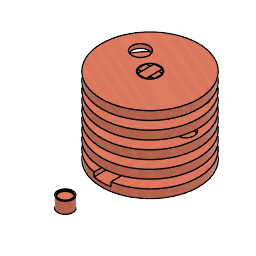
NestorBrinquedo_TorreLabirinto_MariaCarrilho (Autodesk Fusion 360 design; units mm, degrees)
Autodesk Fusion 360 part; units mm, degrees
note: some values were not read from the file. Set by a fixed rule: which sketch regions a step uses; which face or edge a step refers to.
sketch "Esboço1" plane through (0, 0, 0) normal (0, 1, 0) x (1, 0, 0) in component "Camada_2"
  circle A0 centre (0, 0) radius 11.3803
  line L0 (10, 5) -> (-10, 5)
  line L1 (-10, 5) -> (-10, -5)
  line L2 (-10, -5) -> (10, -5)
  line L3 (10, -5) -> (10, 5)
  line L4 (10, 5) -> (-10, -5) construction
  line L5 (-10, 5) -> (10, -5) construction
  line L6 (5, 10) -> (-5, 10)
  line L7 (-5, 10) -> (-5, -10)
  line L8 (-5, -10) -> (5, -10)
  line L9 (5, -10) -> (5, 10)
  line L10 (5, 10) -> (-5, -10) construction
  line L11 (-5, 10) -> (5, -10) construction
  spline S0 degree 3 poles (41.2019, -26.9625) (41.0951, -21.5825) (35.0181, -15.8495) (34.4042, -15.28) knots 0 0 0 0 1 1 1 1
  spline S1 degree 2 poles (34.4042, -15.28) (29.2732, -10.5317) (18.8986, -4.6652) knots 0 0 0 1 1 1
  spline S2 degree 3 poles (18.8986, -4.6652) (18.4699, -4.2135) (17.9685, -3.7052) (17.3893, -2.8657) knots 0 0 0 0 1 1 1 1
  spline S3 degree 3 poles (2.7382, 14.1172) (2.5277, 14.3871) (2.2815, 14.7312) (2.0205, 15.1909) knots 0 0 0 0 1 1 1 1
  spline S4 degree 2 poles (2.0205, 15.1909) (0.8016, 17.3352) (0.4873, 20.138) knots 0 0 0 1 1 1
  spline S5 degree 3 poles (0.4873, 20.138) (0.4873, 20.1409) (0.4873, 20.2892) (0.2856, 21.4578) knots 0 0 0 0 1 1 1 1
  spline S6 degree 3 poles (0.2856, 21.4578) (-0.9393, 28.5165) (0.2885, 39.1461) (4.4259, 42.7141) knots 0 0 0 0 1 1 1 1
  spline S7 degree 3 poles (4.4259, 42.7141) (4.7877, 43.0255) (5.805, 43.8293) (6.2617, 45.2291) knots 0 0 0 0 1 1 1 1
  spline S8 degree 3 poles (6.2617, 45.2291) (6.8045, 46.8841) (6.499, 49.153) (5.2978, 49.7135) knots 0 0 0 0 1 1 1 1
  spline S9 degree 3 poles (5.2978, 49.7135) (4.3962, 50.1347) (3.2603, 49.4674) (2.7502, 49.1619) knots 0 0 0 0 1 1 1 1
  spline S10 degree 3 poles (2.7502, 49.1619) (-1.8558, 46.3799) (-3.7807, 38.2505) (-3.9675, 37.4319) knots 0 0 0 0 1 1 1 1
  spline S11 degree 2 poles (-3.9675, 37.4319) (-5.5157, 30.6164) (-5.4059, 18.6966) knots 0 0 0 1 1 1
  spline S12 degree 3 poles (-5.4059, 18.6966) (-5.4952, 18.0832) (-5.5848, 17.3707) (-5.8856, 16.4) knots 0 0 0 0 1 1 1 1
  spline S13 degree 3 poles (-13.5935, -4.6916) (-13.724, -5.006) (-13.9019, -5.3916) (-14.1689, -5.8454) knots 0 0 0 0 1 1 1 1
  spline S14 degree 2 poles (-14.1689, -5.8454) (-15.4145, -7.9689) (-17.6834, -9.6476) knots 0 0 0 1 1 1
  line L12 (-17.6834, -9.6476) -> (-17.6861, -9.6476)
  spline S15 degree 2 poles (-17.6861, -9.6476) (-17.8166, -9.7217) (-18.7241, -10.481) knots 0 0 0 1 1 1
  spline S16 degree 3 poles (-18.7241, -10.481) (-24.2258, -15.0721) (-34.0457, -19.3222) (-39.2034, -17.5249) knots 0 0 0 0 1 1 1 1
  spline S17 degree 3 poles (-39.2034, -17.5249) (-39.6571, -17.3677) (-40.8583, -16.8872) (-42.3027, -17.1927) knots 0 0 0 0 1 1 1 1
  spline S18 degree 3 poles (-42.3027, -17.1927) (-44.0081, -17.5486) (-45.8172, -18.9485) (-45.7016, -20.2683) knots 0 0 0 0 1 1 1 1
  spline S19 degree 3 poles (-45.7016, -20.2683) (-45.6156, -21.2619) (-44.4707, -21.9114) (-43.9487, -22.1991) knots 0 0 0 0 1 1 1 1
  spline S20 degree 3 poles (-43.9487, -22.1991) (-39.239, -24.7972) (-31.2341, -22.4007) (-30.4333, -22.1516) knots 0 0 0 0 1 1 1 1
  spline S21 degree 2 poles (-30.4333, -22.1516) (-23.7572, -20.0844) (-13.4894, -14.0311) knots 0 0 0 1 1 1
  spline S22 degree 3 poles (-13.4894, -14.0311) (-12.9117, -13.8003) (-12.2543, -13.5185) (-11.2626, -13.2872) knots 0 0 0 0 1 1 1 1
  spline S23 degree 3 poles (10.8582, -9.4283) (11.1963, -9.3809) (11.6175, -9.3423) (12.1484, -9.3453) knots 0 0 0 0 1 1 1 1
  spline S24 degree 2 poles (12.1484, -9.3453) (14.61, -9.3631) (17.1962, -10.4931) knots 0 0 0 1 1 1
  line L13 (17.1962, -10.4931) -> (17.1992, -10.4931)
  spline S25 degree 2 poles (17.1992, -10.4931) (17.3297, -10.5673) (18.4419, -10.9765) knots 0 0 0 1 1 1
  spline S26 degree 3 poles (18.4419, -10.9765) (25.1685, -13.4441) (33.7576, -19.8237) (34.7808, -25.1889) knots 0 0 0 0 1 1 1 1
  spline S27 degree 3 poles (34.7808, -25.1889) (34.8698, -25.6605) (35.0566, -26.9418) (36.0413, -28.0391) knots 0 0 0 0 1 1 1 1
  spline S28 degree 3 poles (36.0413, -28.0391) (37.2039, -29.3352) (39.3216, -30.2042) (40.4071, -29.4449) knots 0 0 0 0 1 1 1 1
  spline S29 degree 3 poles (40.4071, -29.4449) (41.2227, -28.8755) (41.2138, -27.5587) (41.2019, -26.9625) knots 0 0 0 0 1 1 1 1
  circle A1 centre (0, 0) radius 57
  circle A2 centre (0, 0) radius 52
  line L14 (0, 57) -> (0, -57) construction
  circle A3 centre (0, 0) radius 11.1803 construction
  circle A4 centre (0, 0) radius 14.3803
  line L15 (-11.2626, -13.2872) -> (-7.3325, -12.3705)
  line L16 (17.3893, -2.8657) -> (14.2878, 1.6289)
  line L17 (-5.8856, 16.4) -> (-7.0909, 12.5106)
  line L18 (0, -52) -> (45.0333, 26) construction
  line L19 (45.0333, 26) -> (-45.0333, 26) construction
  line L20 (-45.0333, 26) -> (0, -52) construction
  line L21 (0, 0) -> (-45.0333, 26) construction
  line L22 (0, 0) -> (45.0333, 26) construction
  circle A5 centre (0, -31) radius 10
  circle A6 centre (-21.114, 12.1902) radius 10
  circle A7 centre (36.3731, 21) radius 10
  line L23 (0, -14.3803) -> (0, -52) construction
  point P0 (-0.2433, -0.1238)
  dimension "d39" = 10
  dimension "d40" = 10
  dimension "d41" = 20
  dimension "d42" = 20
  dimension "d43" = 0.2
  dimension "d45" = 114
  dimension "d46" = 5
  dimension "d47" = 3
  dimension "d48" = 20
  dimension "d49" = 20
  dimension "d50" = 20
  dimension "d51" = 31
  constraint coincident A0.centre A1.centre
  constraint horizontal L0
  constraint perpendicular L0 L1
  constraint parallel L0 L2
  constraint parallel L1 L3
  constraint coincident L4 A0.centre
  constraint coincident L5 A0.centre
  constraint horizontal L6
  constraint perpendicular L6 L7
  constraint parallel L6 L8
  constraint parallel L7 L9
  constraint coincident L10 A0.centre
  constraint coincident L11 A0.centre
  constraint concentric A0 A1
  constraint concentric A0 A2
  constraint coincident A1 L14.start
  constraint coincident A1 L14.end
  constraint vertical L14
  constraint coincident A0.centre L14
  constraint concentric A1 A3
  constraint coincident L6.start A3
  constraint concentric A0 A4
  constraint coincident S13.start A4
  constraint coincident S3.start A4
  constraint coincident S23.start A4
  constraint coincident A4 L15.end
  constraint coincident A4 L16.end
  constraint coincident A4 L17.end
  constraint coincident L14 L18.start
  constraint coincident A2 L18.start
  constraint coincident L21 A6.centre
  constraint coincident L22 A7.centre
  constraint tangent A2 A7
  constraint tangent A4 A6
  constraint coincident L14 L23.start
  constraint coincident A4 L23.start
  constraint coincident A5.centre L23
  measures "d39" distance of L0 L2
  measures "d40" distance of L7 L9
  measures "d41" distance of L1 L3
  measures "d42" distance of L6 L8
  measures "d43" distance of A0 A3
  measures "d45" diameter of A1
  measures "d46" distance of A1 A2
  measures "d47" distance of A0 A4
  measures "d48" diameter of A6
  measures "d49" diameter of A7
  measures "d50" diameter of A5
  measures "d51" distance of A0.centre A5.centre
sketch "Esboço1 (2)" plane through (0, 0, 0) normal (0, 1, 0) x (1, 0, 0) in component "Camada_3"
  line L0 (-5, 10) -> (-5, -10)
  line L1 (5, 10) -> (-5, 10)
  line L2 (-5, 10) -> (5, -10) construction
  line L3 (5, 10) -> (-5, -10) construction
  line L4 (5, -10) -> (5, 10)
  line L5 (-5, -10) -> (5, -10)
  line L6 (-10, -5) -> (10, -5)
  line L7 (-10, 5) -> (10, -5) construction
  line L8 (10, -5) -> (10, 5)
  line L9 (10, 5) -> (-10, -5) construction
  line L10 (10, 5) -> (-10, 5)
  line L11 (-10, 5) -> (-10, -5)
  circle A0 centre (0, 0) radius 11.1803 construction
  circle A1 centre (0, 0) radius 11.3803
  circle A2 centre (0, 0) radius 14.3803
  circle A3 centre (0, 0) radius 57
  circle A4 centre (0, 0) radius 52
  line L12 (-5.8856, 16.4) -> (-7.0909, 12.5106)
  spline S0 degree 3 poles (-5.4059, 18.6966) (-5.4952, 18.0832) (-5.5848, 17.3707) (-5.8856, 16.4) knots 0 0 0 0 1 1 1 1
  spline S1 degree 2 poles (-3.9675, 37.4319) (-5.5157, 30.6164) (-5.4059, 18.6966) knots 0 0 0 1 1 1
  spline S2 degree 3 poles (0.4873, 20.138) (0.4873, 20.1409) (0.4873, 20.2892) (0.2856, 21.4578) knots 0 0 0 0 1 1 1 1
  spline S3 degree 2 poles (2.0205, 15.1909) (0.8016, 17.3352) (0.4873, 20.138) knots 0 0 0 1 1 1
  spline S4 degree 3 poles (2.7382, 14.1172) (2.5277, 14.3871) (2.2815, 14.7312) (2.0205, 15.1909) knots 0 0 0 0 1 1 1 1
  spline S5 degree 3 poles (0.2856, 21.4578) (-0.9393, 28.5165) (0.2885, 39.1461) (4.4259, 42.7141) knots 0 0 0 0 1 1 1 1
  spline S6 degree 3 poles (2.7502, 49.1619) (-1.8558, 46.3799) (-3.7807, 38.2505) (-3.9675, 37.4319) knots 0 0 0 0 1 1 1 1
  spline S7 degree 3 poles (5.2978, 49.7135) (4.3962, 50.1347) (3.2603, 49.4674) (2.7502, 49.1619) knots 0 0 0 0 1 1 1 1
  spline S8 degree 3 poles (6.2617, 45.2291) (6.8045, 46.8841) (6.499, 49.153) (5.2978, 49.7135) knots 0 0 0 0 1 1 1 1
  spline S9 degree 3 poles (4.4259, 42.7141) (4.7877, 43.0255) (5.805, 43.8293) (6.2617, 45.2291) knots 0 0 0 0 1 1 1 1
  line L13 (0, -14.3803) -> (0, -52) construction
  line L14 (0, 57) -> (0, -57) construction
  spline S10 degree 3 poles (-6.262, -45.2316) (-6.8065, -46.8864) (-6.4987, -49.1531) (-5.2979, -49.7129) knots 0 0 0 0 1 1 1 1
  line L15 (-6.262, -45.2316) -> (-6.8065, -46.8864) construction
  line L16 (-6.8065, -46.8864) -> (-6.4987, -49.1531) construction
  line L17 (-6.4987, -49.1531) -> (-5.2979, -49.7129) construction
  spline S11 degree 3 poles (-5.2979, -49.7129) (-4.3945, -50.1352) (-3.2596, -49.4685) (-2.7494, -49.1603) knots 0 0 0 0 1 1 1 1
  line L18 (-5.2979, -49.7129) -> (-4.3945, -50.1352) construction
  line L19 (-4.3945, -50.1352) -> (-3.2596, -49.4685) construction
  line L20 (-3.2596, -49.4685) -> (-2.7494, -49.1603) construction
  spline S12 degree 3 poles (-2.7494, -49.1603) (1.8555, -46.3805) (3.7826, -38.2499) (3.9672, -37.4318) knots 0 0 0 0 1 1 1 1
  line L21 (-2.7494, -49.1603) -> (1.8555, -46.3805) construction
  line L22 (1.8555, -46.3805) -> (3.7826, -38.2499) construction
  line L23 (3.7826, -38.2499) -> (3.9672, -37.4318) construction
  spline S13 degree 3 poles (-4.4247, -42.7135) (-4.7877, -43.0279) (-5.8044, -43.8279) (-6.262, -45.2316) knots 0 0 0 0 1 1 1 1
  line L24 (-4.4247, -42.7135) -> (-4.7877, -43.0279) construction
  line L25 (-4.7877, -43.0279) -> (-5.8044, -43.8279) construction
  line L26 (-5.8044, -43.8279) -> (-6.262, -45.2316) construction
  spline S14 degree 3 poles (-0.2852, -21.456) (0.94, -28.5162) (-0.2894, -39.1456) (-4.4247, -42.7135) knots 0 0 0 0 1 1 1 1
  line L27 (-0.2852, -21.456) -> (0.94, -28.5162) construction
  line L28 (0.94, -28.5162) -> (-0.2894, -39.1456) construction
  line L29 (-0.2894, -39.1456) -> (-4.4247, -42.7135) construction
  spline S15 degree 2 poles (3.9672, -37.4318) (5.515, -30.6165) (5.4066, -18.6977) knots 0 0 0 1 1 1
  line L30 (3.9672, -37.4318) -> (5.515, -30.6165) construction
  line L31 (5.515, -30.6165) -> (5.4066, -18.6977) construction
  spline S16 degree 2 poles (-2.0222, -15.1933) (-0.806, -17.3338) (-0.4867, -20.1381) knots 0 0 0 1 1 1
  line L32 (-2.0222, -15.1933) -> (-0.806, -17.3338) construction
  line L33 (-0.806, -17.3338) -> (-0.4867, -20.1381) construction
  spline S17 degree 2 poles (-0.4867, -20.1381) (-0.4878, -20.2976) (-0.2852, -21.456) knots 0 0 0 1 1 1
  line L34 (-0.4867, -20.1381) -> (-0.4878, -20.2976) construction
  line L35 (-0.4878, -20.2976) -> (-0.2852, -21.456) construction
  spline S18 degree 3 poles (5.4066, -18.6977) (5.4956, -18.082) (5.5803, -17.3718) (5.8758, -16.3973) knots 0 0 0 0 1 1 1 1
  line L36 (5.4066, -18.6977) -> (5.4956, -18.082) construction
  line L37 (5.4956, -18.082) -> (5.5803, -17.3718) construction
  line L38 (5.5803, -17.3718) -> (5.8758, -16.3973) construction
  line L39 (5.8758, -16.3973) -> (7.0469, -12.5353)
  spline S19 degree 3 poles (-2.7337, -14.1181) (-2.5266, -14.3883) (-2.2817, -14.7352) (-2.0222, -15.1933) knots 0 0 0 0 1 1 1 1
  line L40 (-2.7337, -14.1181) -> (-2.5266, -14.3883) construction
  line L41 (-2.5266, -14.3883) -> (-2.2817, -14.7352) construction
  line L42 (-2.2817, -14.7352) -> (-2.0222, -15.1933) construction
  line L43 (-57, 0) -> (57, 0) construction
  circle A5 centre (-24.3803, 0) radius 10
  circle A6 centre (42, 0) radius 10
  dimension "d52" = 20
  dimension "d53" = 20
  constraint coincident A3 L43.start
  constraint coincident A3 L43.end
  constraint perpendicular L8 L43
  constraint coincident L43 A0.centre
  constraint coincident L43 A5.centre
  constraint coincident L43 A6.centre
  constraint tangent A2 A5
  constraint tangent A4 A6
  constraint coincident A2 S19.start
  constraint coincident A2 L39.end
  constraint coincident S16.end L33.end
  measures "d52" diameter of A5
  measures "d53" diameter of A6
sketch "Esboço1 (3)" plane through (0, 0, 0) normal (0, 1, 0) x (1, 0, 0) in component "Camada_4"
  circle A0 centre (0, 0) radius 57
  circle A1 centre (0, 0) radius 52
  line L0 (-5.8856, 16.4) -> (-7.0909, 12.5106)
  spline S0 degree 3 poles (-5.4059, 18.6966) (-5.4952, 18.0832) (-5.5848, 17.3707) (-5.8856, 16.4) knots 0 0 0 0 1 1 1 1
  spline S1 degree 2 poles (-3.9675, 37.4319) (-5.5157, 30.6164) (-5.4059, 18.6966) knots 0 0 0 1 1 1
  spline S2 degree 3 poles (2.7502, 49.1619) (-1.8558, 46.3799) (-3.7807, 38.2505) (-3.9675, 37.4319) knots 0 0 0 0 1 1 1 1
  spline S3 degree 3 poles (5.2978, 49.7135) (4.3962, 50.1347) (3.2603, 49.4674) (2.7502, 49.1619) knots 0 0 0 0 1 1 1 1
  spline S4 degree 3 poles (6.2617, 45.2291) (6.8045, 46.8841) (6.499, 49.153) (5.2978, 49.7135) knots 0 0 0 0 1 1 1 1
  spline S5 degree 3 poles (4.4259, 42.7141) (4.7877, 43.0255) (5.805, 43.8293) (6.2617, 45.2291) knots 0 0 0 0 1 1 1 1
  spline S6 degree 3 poles (0.2856, 21.4578) (-0.9393, 28.5165) (0.2885, 39.1461) (4.4259, 42.7141) knots 0 0 0 0 1 1 1 1
  spline S7 degree 2 poles (2.0205, 15.1909) (0.8016, 17.3352) (0.4873, 20.138) knots 0 0 0 1 1 1
  spline S8 degree 3 poles (0.4873, 20.138) (0.4873, 20.1409) (0.4873, 20.2892) (0.2856, 21.4578) knots 0 0 0 0 1 1 1 1
  spline S9 degree 3 poles (2.7382, 14.1172) (2.5277, 14.3871) (2.2815, 14.7312) (2.0205, 15.1909) knots 0 0 0 0 1 1 1 1
  circle A2 centre (0, 0) radius 14.3803
  circle A3 centre (0, 0) radius 11.3803
  circle A4 centre (0, 0) radius 11.1803 construction
  line L1 (10, 5) -> (-10, -5) construction
  line L2 (-10, 5) -> (-10, -5)
  line L3 (-10, 5) -> (10, -5) construction
  line L4 (10, 5) -> (-10, 5)
  line L5 (-5, 10) -> (-5, -10)
  line L6 (5, 10) -> (-5, 10)
  line L7 (-5, 10) -> (5, -10) construction
  line L8 (5, 10) -> (-5, -10) construction
  line L9 (5, -10) -> (5, 10)
  line L10 (-10, -5) -> (10, -5)
  line L11 (-5, -10) -> (5, -10)
  line L12 (10, -5) -> (10, 5)
  line L13 (0, 57) -> (0, -57) construction
  circle A5 centre (0, -31) radius 10
sketch "Esboço1 (4)" plane through (0, 0, 0) normal (0, 1, 0) x (1, 0, 0) in component "Base"
  circle A0 centre (0, 0) radius 57
  circle A1 centre (0, 0) radius 52
  circle A2 centre (0, 0) radius 14.3803
  circle A3 centre (0, 0) radius 11.3803
  circle A4 centre (0, 0) radius 11.1803 construction
  line L0 (-10, -5) -> (10, -5)
  line L1 (-10, 5) -> (-10, -5)
  line L2 (10, 5) -> (-10, -5) construction
  line L3 (-10, 5) -> (10, -5) construction
  line L4 (10, 5) -> (-10, 5)
  line L5 (-5, 10) -> (-5, -10)
  line L6 (5, 10) -> (-5, 10)
  line L7 (5, -10) -> (5, 10)
  line L8 (5, 10) -> (-5, -10) construction
  line L9 (-5, 10) -> (5, -10) construction
  line L10 (10, -5) -> (10, 5)
  line L11 (-5, -10) -> (5, -10)
  circle A5 centre (0, -31) radius 10
  line L12 (0, 57) -> (0, -57) construction
  line L13 (-10, -31) -> (10, -31) construction
  line L14 (-10, -31) -> (10, -31) construction
  line L15 (10, -31) -> (10, -57)
  line L16 (10, -57) -> (-10, -57)
  line L17 (-10, -57) -> (-10, -31)
  constraint coincident A5 L13.start
  constraint coincident A5 L13.end
  constraint perpendicular L12 L13
  constraint perpendicular L14 L15
  constraint parallel L14 L16
  constraint parallel L15 L17
  constraint coincident L12.end L16
  constraint tangent A5 L17
sketch "Esboço1 (5)" plane through (0, 0, 0) normal (0, 1, 0) x (1, 0, 0) in component "Tampa_cam1"
  circle A0 centre (0, 0) radius 57
  circle A1 centre (0, 0) radius 52
  spline S0 degree 3 poles (5.2978, 49.7135) (4.3962, 50.1347) (3.2603, 49.4674) (2.7502, 49.1619) knots 0 0 0 0 1 1 1 1
  spline S1 degree 3 poles (6.2617, 45.2291) (6.8045, 46.8841) (6.499, 49.153) (5.2978, 49.7135) knots 0 0 0 0 1 1 1 1
  spline S2 degree 3 poles (4.4259, 42.7141) (4.7877, 43.0255) (5.805, 43.8293) (6.2617, 45.2291) knots 0 0 0 0 1 1 1 1
  spline S3 degree 3 poles (0.2856, 21.4578) (-0.9393, 28.5165) (0.2885, 39.1461) (4.4259, 42.7141) knots 0 0 0 0 1 1 1 1
  spline S4 degree 3 poles (2.7502, 49.1619) (-1.8558, 46.3799) (-3.7807, 38.2505) (-3.9675, 37.4319) knots 0 0 0 0 1 1 1 1
  spline S5 degree 2 poles (-3.9675, 37.4319) (-5.5157, 30.6164) (-5.4059, 18.6966) knots 0 0 0 1 1 1
  spline S6 degree 3 poles (-5.4059, 18.6966) (-5.4952, 18.0832) (-5.5848, 17.3707) (-5.8856, 16.4) knots 0 0 0 0 1 1 1 1
  line L0 (-5.8856, 16.4) -> (-7.0909, 12.5106)
  spline S7 degree 2 poles (2.0205, 15.1909) (0.8016, 17.3352) (0.4873, 20.138) knots 0 0 0 1 1 1
  spline S8 degree 3 poles (0.4873, 20.138) (0.4873, 20.1409) (0.4873, 20.2892) (0.2856, 21.4578) knots 0 0 0 0 1 1 1 1
  spline S9 degree 3 poles (2.7382, 14.1172) (2.5277, 14.3871) (2.2815, 14.7312) (2.0205, 15.1909) knots 0 0 0 0 1 1 1 1
  circle A2 centre (0, 0) radius 14.3803
  circle A3 centre (0, 0) radius 11.3803
  circle A4 centre (0, 0) radius 11.1803 construction
  line L1 (5, 10) -> (-5, 10)
  line L2 (-5, 10) -> (-5, -10)
  line L3 (-5, -10) -> (5, -10)
  line L4 (5, -10) -> (5, 10)
  line L5 (10, 5) -> (-10, 5)
  line L6 (-10, 5) -> (-10, -5)
  line L7 (-10, -5) -> (10, -5)
  line L8 (10, -5) -> (10, 5)
  line L9 (-10, 5) -> (10, -5) construction
  line L10 (10, 5) -> (-10, -5) construction
  line L11 (5, 10) -> (-5, -10) construction
  line L12 (-5, 10) -> (5, -10) construction
  line L13 (0, 57) -> (0, -57) construction
  line L14 (-57, 0) -> (57, 0) construction
  spline S10 degree 3 poles (-5.2979, -49.7129) (-4.3945, -50.1352) (-3.2596, -49.4685) (-2.7494, -49.1603) knots 0 0 0 0 1 1 1 1
  spline S11 degree 3 poles (-6.262, -45.2316) (-6.8065, -46.8864) (-6.4987, -49.1531) (-5.2979, -49.7129) knots 0 0 0 0 1 1 1 1
  spline S12 degree 3 poles (-4.4247, -42.7135) (-4.7877, -43.0279) (-5.8044, -43.8279) (-6.262, -45.2316) knots 0 0 0 0 1 1 1 1
  spline S13 degree 3 poles (-0.2852, -21.456) (0.94, -28.5162) (-0.2894, -39.1456) (-4.4247, -42.7135) knots 0 0 0 0 1 1 1 1
  spline S14 degree 3 poles (-2.7494, -49.1603) (1.8555, -46.3805) (3.7826, -38.2499) (3.9672, -37.4318) knots 0 0 0 0 1 1 1 1
  spline S15 degree 2 poles (3.9672, -37.4318) (5.515, -30.6165) (5.4066, -18.6977) knots 0 0 0 1 1 1
  spline S16 degree 2 poles (-0.4867, -20.1381) (-0.4878, -20.2976) (-0.2852, -21.456) knots 0 0 0 1 1 1
  spline S17 degree 2 poles (-2.0222, -15.1933) (-0.806, -17.3338) (-0.4867, -20.1381) knots 0 0 0 1 1 1
  spline S18 degree 3 poles (5.4066, -18.6977) (5.4956, -18.082) (5.5803, -17.3718) (5.8758, -16.3973) knots 0 0 0 0 1 1 1 1
  line L15 (5.8758, -16.3973) -> (7.0469, -12.5353)
  spline S19 degree 3 poles (-2.7337, -14.1181) (-2.5266, -14.3883) (-2.2817, -14.7352) (-2.0222, -15.1933) knots 0 0 0 0 1 1 1 1
  spline S20 degree 2 poles (-37.4319, -3.9675) (-30.6164, -5.5157) (-18.6966, -5.4059) knots 0 0 0 1 1 1
  line L16 (-37.4319, -3.9675) -> (-30.6164, -5.5157) construction
  line L17 (-30.6164, -5.5157) -> (-18.6966, -5.4059) construction
  spline S21 degree 3 poles (-18.6966, -5.4059) (-18.0832, -5.4952) (-17.3707, -5.5848) (-16.4, -5.8856) knots 0 0 0 0 1 1 1 1
  line L18 (-18.6966, -5.4059) -> (-18.0832, -5.4952) construction
  line L19 (-18.0832, -5.4952) -> (-17.3707, -5.5848) construction
  line L20 (-17.3707, -5.5848) -> (-16.4, -5.8856) construction
  line L21 (-16.4, -5.8856) -> (-12.5106, -7.0909)
  spline S22 degree 2 poles (-15.1909, 2.0205) (-17.3352, 0.8016) (-20.138, 0.4873) knots 0 0 0 1 1 1
  line L22 (-15.1909, 2.0205) -> (-17.3352, 0.8016) construction
  line L23 (-17.3352, 0.8016) -> (-20.138, 0.4873) construction
  spline S23 degree 3 poles (-14.1172, 2.7382) (-14.3871, 2.5277) (-14.7312, 2.2815) (-15.1909, 2.0205) knots 0 0 0 0 1 1 1 1
  line L24 (-14.1172, 2.7382) -> (-14.3871, 2.5277) construction
  line L25 (-14.3871, 2.5277) -> (-14.7312, 2.2815) construction
  line L26 (-14.7312, 2.2815) -> (-15.1909, 2.0205) construction
  spline S24 degree 3 poles (-21.4578, 0.2856) (-28.5165, -0.9393) (-39.1461, 0.2885) (-42.7141, 4.4259) knots 0 0 0 0 1 1 1 1
  line L27 (-21.4578, 0.2856) -> (-28.5165, -0.9393) construction
  line L28 (-28.5165, -0.9393) -> (-39.1461, 0.2885) construction
  line L29 (-39.1461, 0.2885) -> (-42.7141, 4.4259) construction
  spline S25 degree 3 poles (-20.138, 0.4873) (-20.1409, 0.4873) (-20.2892, 0.4873) (-21.4578, 0.2856) knots 0 0 0 0 1 1 1 1
  line L30 (-20.138, 0.4873) -> (-20.1409, 0.4873) construction
  line L31 (-20.1409, 0.4873) -> (-20.2892, 0.4873) construction
  line L32 (-20.2892, 0.4873) -> (-21.4578, 0.2856) construction
  spline S26 degree 3 poles (-49.1619, 2.7502) (-46.3799, -1.8558) (-38.2505, -3.7807) (-37.4319, -3.9675) knots 0 0 0 0 1 1 1 1
  line L33 (-49.1619, 2.7502) -> (-46.3799, -1.8558) construction
  line L34 (-46.3799, -1.8558) -> (-38.2505, -3.7807) construction
  line L35 (-38.2505, -3.7807) -> (-37.4319, -3.9675) construction
  spline S27 degree 3 poles (-49.7135, 5.2978) (-50.1347, 4.3962) (-49.4674, 3.2603) (-49.1619, 2.7502) knots 0 0 0 0 1 1 1 1
  line L36 (-49.7135, 5.2978) -> (-50.1347, 4.3962) construction
  line L37 (-50.1347, 4.3962) -> (-49.4674, 3.2603) construction
  line L38 (-49.4674, 3.2603) -> (-49.1619, 2.7502) construction
  spline S28 degree 3 poles (-45.2291, 6.2617) (-46.8841, 6.8045) (-49.153, 6.499) (-49.7135, 5.2978) knots 0 0 0 0 1 1 1 1
  line L39 (-45.2291, 6.2617) -> (-46.8841, 6.8045) construction
  line L40 (-46.8841, 6.8045) -> (-49.153, 6.499) construction
  line L41 (-49.153, 6.499) -> (-49.7135, 5.2978) construction
  spline S29 degree 3 poles (-42.7141, 4.4259) (-43.0255, 4.7877) (-43.8293, 5.805) (-45.2291, 6.2617) knots 0 0 0 0 1 1 1 1
  line L42 (-42.7141, 4.4259) -> (-43.0255, 4.7877) construction
  line L43 (-43.0255, 4.7877) -> (-43.8293, 5.805) construction
  line L44 (-43.8293, 5.805) -> (-45.2291, 6.2617) construction
  spline S30 degree 3 poles (20.138, -0.4873) (20.1409, -0.4873) (20.2892, -0.4873) (21.4578, -0.2856) knots 0 0 0 0 1 1 1 1
  line L45 (20.138, -0.4873) -> (20.1409, -0.4873) construction
  line L46 (20.1409, -0.4873) -> (20.2892, -0.4873) construction
  line L47 (20.2892, -0.4873) -> (21.4578, -0.2856) construction
  spline S31 degree 2 poles (15.1909, -2.0205) (17.3352, -0.8016) (20.138, -0.4873) knots 0 0 0 1 1 1
  line L48 (15.1909, -2.0205) -> (17.3352, -0.8016) construction
  line L49 (17.3352, -0.8016) -> (20.138, -0.4873) construction
  spline S32 degree 3 poles (45.2291, -6.2617) (46.8841, -6.8045) (49.153, -6.499) (49.7135, -5.2978) knots 0 0 0 0 1 1 1 1
  line L50 (45.2291, -6.2617) -> (46.8841, -6.8045) construction
  line L51 (46.8841, -6.8045) -> (49.153, -6.499) construction
  line L52 (49.153, -6.499) -> (49.7135, -5.2978) construction
  spline S33 degree 3 poles (49.7135, -5.2978) (50.1347, -4.3962) (49.4674, -3.2603) (49.1619, -2.7502) knots 0 0 0 0 1 1 1 1
  line L53 (49.7135, -5.2978) -> (50.1347, -4.3962) construction
  line L54 (50.1347, -4.3962) -> (49.4674, -3.2603) construction
  line L55 (49.4674, -3.2603) -> (49.1619, -2.7502) construction
  spline S34 degree 3 poles (42.7141, -4.4259) (43.0255, -4.7877) (43.8293, -5.805) (45.2291, -6.2617) knots 0 0 0 0 1 1 1 1
  line L56 (42.7141, -4.4259) -> (43.0255, -4.7877) construction
  line L57 (43.0255, -4.7877) -> (43.8293, -5.805) construction
  line L58 (43.8293, -5.805) -> (45.2291, -6.2617) construction
  line L59 (16.4, 5.8856) -> (12.5106, 7.0909)
  spline S35 degree 2 poles (37.4319, 3.9675) (30.6164, 5.5157) (18.6966, 5.4059) knots 0 0 0 1 1 1
  line L60 (37.4319, 3.9675) -> (30.6164, 5.5157) construction
  line L61 (30.6164, 5.5157) -> (18.6966, 5.4059) construction
  spline S36 degree 3 poles (49.1619, -2.7502) (46.3799, 1.8558) (38.2505, 3.7807) (37.4319, 3.9675) knots 0 0 0 0 1 1 1 1
  line L62 (49.1619, -2.7502) -> (46.3799, 1.8558) construction
  line L63 (46.3799, 1.8558) -> (38.2505, 3.7807) construction
  line L64 (38.2505, 3.7807) -> (37.4319, 3.9675) construction
  spline S37 degree 3 poles (14.1172, -2.7382) (14.3871, -2.5277) (14.7312, -2.2815) (15.1909, -2.0205) knots 0 0 0 0 1 1 1 1
  line L65 (14.1172, -2.7382) -> (14.3871, -2.5277) construction
  line L66 (14.3871, -2.5277) -> (14.7312, -2.2815) construction
  line L67 (14.7312, -2.2815) -> (15.1909, -2.0205) construction
  spline S38 degree 3 poles (18.6966, 5.4059) (18.0832, 5.4952) (17.3707, 5.5848) (16.4, 5.8856) knots 0 0 0 0 1 1 1 1
  line L68 (18.6966, 5.4059) -> (18.0832, 5.4952) construction
  line L69 (18.0832, 5.4952) -> (17.3707, 5.5848) construction
  line L70 (17.3707, 5.5848) -> (16.4, 5.8856) construction
  spline S39 degree 3 poles (21.4578, -0.2856) (28.5165, 0.9393) (39.1461, -0.2885) (42.7141, -4.4259) knots 0 0 0 0 1 1 1 1
  line L71 (21.4578, -0.2856) -> (28.5165, 0.9393) construction
  line L72 (28.5165, 0.9393) -> (39.1461, -0.2885) construction
  line L73 (39.1461, -0.2885) -> (42.7141, -4.4259) construction
  line L74 (0, 0) -> (-45.0333, 26) construction
  circle A5 centre (-26.8468, 15.5) radius 10
  circle A6 centre (0, 0) radius 57
  dimension "d54" = 20
  dimension "d55" = 31
  constraint coincident L74 A5.centre
  measures "d54" diameter of A5
  measures "d55" distance of A5.centre A0.centre
extrude "Extrusão1" add sketch "Esboço1 (4)" along normal blind 10 contours A0 A1 L15 L17 | A1 A5 L15 L17 | A2 | A3 picked at (-12.6917, -53.7345) picked at (-20.779, -22.0556) makes body 1 in component "Base"
extrude "Extrusão2" add sketch "Esboço1 (4)" along normal blind 5 contours A0 A1 L15 L17 | A1 A5 L15 L17 | A5 picked at (0, -53.5946) picked at (5.6684, -47.7433) bodies 1 in component "Base"
extrude "Extrusão1'" add sketch "Esboço1 (3)" along normal blind 20 from surface at 10 separate body contours A2 makes body 2 in component "Camada_4"
extrude "Extrusão2'" add sketch "Esboço1 (3)" against normal blind 5 from surface at 30 contours A1 bodies 2 in component "Camada_4"
extrude "Extrusão3" add sketch "Esboço1 (3)" against normal blind 10 from surface at 30 contours A0 bodies 2 in component "Camada_4"
extrude "Extrusão4" add sketch "Esboço1 (3)" against normal blind 8 from surface at 30 contours L0 S0 S1 S2 S3 S4 S5 S6 S7 S8 S9 A2 bodies 2 in component "Camada_4"
extrude "Extrusão1''" add sketch "Esboço1 (2)" along normal blind 20 from surface at 30 separate body contours A2 makes body 3 in component "Camada_3"
extrude "Extrusão2''" add sketch "Esboço1 (2)" against normal blind 5 from surface at 50 contours A2 L12 S0 S1 S2 S3 S4 S5 S6 S7 S8 S9 | A2 S10 S11 S12 S13 S14 S15 S16 S17 S18 L39 S19 | A4 bodies 3 in component "Camada_3"
extrude "Extrusão3'" add sketch "Esboço1 (2)" against normal blind 10 from surface at 50 contours A3 bodies 3 in component "Camada_3"
extrude "Extrusão4'" add sketch "Esboço1 (2)" against normal blind 3 from surface at 45 contours A2 L12 S0 S1 S2 S3 S4 S5 S6 S7 S8 S9 | A2 S10 S11 S12 S13 S14 S15 S16 S17 S18 L39 S19 bodies 3 in component "Camada_3"
extrude "Extrusão5" add sketch "Esboço1" along normal blind 20 from surface at 50 separate body contours A4 makes body 4 in component "Camada_2"
extrude "Extrusão6" add sketch "Esboço1" against normal blind 5 from surface at 70 contours S0 S1 S2 S23 S24 L13 S25 S26 S27 S28 S29 A4 L16 | S3 S4 S5 S6 S7 S8 S9 S10 S11 S12 A4 L17 | S13 S14 L12 S15 S16 S17 S18 S19 S20 S21 S22 A4 L15 | A1 | A2 bodies 4 in component "Camada_2"
extrude "Extrusão7" add sketch "Esboço1" against normal blind 5 from surface at 65 contours A1 bodies 4 in component "Camada_2"
extrude "Extrusão8" add sketch "Esboço1" against normal blind 3 from surface at 65 contours S0 S1 S2 S23 S24 L13 S25 S26 S27 S28 S29 A4 L16 | S3 S4 S5 S6 S7 S8 S9 S10 S11 S12 A4 L17 | S13 S14 L12 S15 S16 S17 S18 S19 S20 S21 S22 A4 L15 bodies 4 in component "Camada_2"
extrude "Extrusão1'''" add sketch "Esboço1 (5)" along normal blind 20 from surface at 70 separate body contours A2 makes body 5 in component "Tampa_cam1"
extrude "Extrusão2'''" add sketch "Esboço1 (5)" against normal blind 5 from surface at 90 contours A0 A6 | A1 | S0 S1 S2 S3 S4 S5 S6 L0 S7 S8 S9 A2 | A2 S20 S21 L21 S22 S23 S24 S25 S26 S27 S28 S29 | A2 S30 S31 S32 S33 S34 L59 S35 S36 S37 S38 S39 | A2 S10 S11 S12 S13 S14 S15 S16 S17 S18 L15 S19 bodies 5 in component "Tampa_cam1"
extrude "Extrusão3''" add sketch "Esboço1 (5)" against normal blind 5 from surface at 85 contours A0 A6 bodies 5 in component "Tampa_cam1"
extrude "Extrusão4''" add sketch "Esboço1 (5)" against normal blind 3 from surface at 85 contours S0 S1 S2 S3 S4 S5 S6 L0 S7 S8 S9 A2 | A2 S20 S21 L21 S22 S23 S24 S25 S26 S27 S28 S29 | A2 S30 S31 S32 S33 S34 L59 S35 S36 S37 S38 S39 | A2 S10 S11 S12 S13 S14 S15 S16 S17 S18 L15 S19 bodies 5 in component "Tampa_cam1"
sketch "Esboço1 (6)" plane through (0, 0, 0) normal (0, 1, 0) x (1, 0, 0) in component "Eixo_1"
  line L0 (10, 5) -> (-10, 5) construction
  line L1 (-10, 5) -> (-10, -5) construction
  line L2 (-10, -5) -> (10, -5) construction
  line L3 (-5, 10) -> (-5, -10) construction
  line L4 (5, -10) -> (5, 10) construction
  line L5 (-5, -10) -> (5, -10) construction
  line L6 (10, -5) -> (10, 5) construction
  line L7 (5, 10) -> (-5, 10) construction
  line L8 (-10, 5) -> (10, -5) construction
  line L9 (-5, 10) -> (5, -10) construction
  line L10 (5, 10) -> (-5, -10) construction
  line L11 (10, 5) -> (-10, -5) construction
extrude "Extrusão1''''" add sketch "Esboço1" along normal up to surface (90 mm away) separate body contours L0 L2 L3 L9 | L0 L2 L7 L9 | L0 L1 L2 L7 makes body 6 in component "Eixo_1"
sketch "Esboço1 (7)" plane through (0, 0, 0) normal (0, 1, 0) x (1, 0, 0) in component "Eixo_2"
  line L0 (-10, 5) -> (-10, -5)
  line L1 (10, 5) -> (-10, 5)
  line L2 (-10, -5) -> (10, -5)
  line L3 (-5, 10) -> (-5, -10)
  line L4 (5, -10) -> (5, 10)
  line L5 (-5, -10) -> (5, -10)
  line L6 (10, -5) -> (10, 5)
  line L7 (5, 10) -> (-5, 10)
  line L8 (-10, 5) -> (10, -5) construction
  line L9 (-5, 10) -> (5, -10) construction
  line L10 (5, 10) -> (-5, -10) construction
  line L11 (10, 5) -> (-10, -5) construction
extrude "Extrusão1'''''" add sketch "Esboço1 (7)" along normal up to surface (90 mm away) separate body contours L1 L3 L4 L7 | L1 L2 L3 L4 | L2 L3 L4 L5 makes body 7 in component "Eixo_2"
sketch "Esboço2" plane through (0, 0, 5) normal (0, 0, 1) x (1, 0, 0) in component "Eixo_1"
  line L0 (10, 90) -> (-10, 90)
  line L1 (-10, 90) -> (-10, 0)
  line L2 (-10, 0) -> (10, 0)
  line L3 (10, 0) -> (10, 90)
  line L4 (0, 90) -> (0, 0) construction
  line L5 (5, 90) -> (-5, 90)
  line L6 (-5, 90) -> (-5, 45)
  line L7 (-5, 45) -> (5, 45)
  line L8 (5, 45) -> (5, 90)
  line L9 (5, 90) -> (-5, 45) construction
  line L10 (-5, 90) -> (5, 45) construction
  circle A0 centre (-5, 45) radius 1.5
  circle A1 centre (5, 45) radius 1.5
  point P0 (0, 67.5)
  dimension "d112" = 10
  dimension "d113" = 45
  dimension "d117" = 3
  dimension "d118" = 3
  constraint midpoint L0 L4.start
  constraint coincident L4.end origin
  constraint horizontal L5
  constraint perpendicular L5 L6
  constraint parallel L5 L7
  constraint parallel L6 L8
  constraint coincident L9 P0
  constraint coincident L10 P0
  constraint coincident L4 P0
  constraint collinear L0 L5
  constraint coincident L6.end L7.start
  constraint coincident L7.end L8.start
  measures "d112" distance of L6.end L7.end
  measures "d113" distance of L5.end L6.end
  measures "d117" diameter of A0
  measures "d118" diameter of A1
extrude "Extrusão2''''" cut sketch "Esboço2" against normal up to surface (10 mm away) contours L0 L5 L6 L7 L8 A0 A1 | L7 L8 A1 | L7 L8 A1 | L6 L7 A0 | L6 L7 A0 bodies 6 in component "Eixo_1"
sketch "Esboço2 (2)" plane through (-5, 0, 0) normal (-1, 0, 0) x (0, 0, 1) in component "Eixo_2"
  line L0 (10, 90) -> (-10, 90)
  line L1 (-10, 90) -> (-10, 0)
  line L2 (-10, 0) -> (10, 0)
  line L3 (10, 0) -> (10, 90)
  line L4 (0, 90) -> (0, 0) construction
  line L5 (5, 45) -> (-5, 45)
  line L6 (-5, 45) -> (-5, 0)
  line L7 (-5, 0) -> (5, 0)
  line L8 (5, 0) -> (5, 45)
  line L9 (5, 45) -> (-5, 0) construction
  line L10 (-5, 45) -> (5, 0) construction
  circle A0 centre (-5, 45) radius 1.5
  circle A1 centre (5, 45) radius 1.5
  point P0 (0, 22.5)
  dimension "d119" = 10
  dimension "d120" = 45
  dimension "d121" = 3
  dimension "d122" = 3
  constraint midpoint L0 L4.start
  constraint coincident L4.end origin
  constraint horizontal L5
  constraint perpendicular L5 L6
  constraint parallel L5 L7
  constraint parallel L6 L8
  constraint coincident L9 P0
  constraint coincident L10 P0
  constraint coincident L4 P0
  constraint collinear L2 L7
  constraint coincident L5.end L6.start
  constraint coincident L5.start L8.end
  measures "d119" distance of L6.end L7.end
  measures "d120" distance of L5.end L6.end
  measures "d121" diameter of A0
  measures "d122" diameter of A1
extrude "Extrusão2'''''" cut sketch "Esboço2 (2)" against normal up to surface (10 mm away) contours L2 L5 L6 L7 L8 A0 A1 | L5 L8 A1 | L5 L8 A1 | L5 L6 A0 | L5 L6 A0 bodies 7 in component "Eixo_2"
sketch "Esboço1 (8)" plane through (0, 0, 0) normal (0, 1, 0) x (1, 0, 0) in component "Peça_Disco"
  circle A0 centre (0, 0) radius 9
  circle A1 centre (0, 0) radius 7.5
  spline S0 degree 3 poles (38.093, -2.5986) (39.5165, -2.6401) (40.7504, -1.4892) (40.7756, -0.0588) knots 2 2 2 2 3 3 3 3
  spline S1 degree 3 poles (40.7756, -0.0588) (40.8001, 1.325) (39.6849, 2.4813) (38.3394, 2.5678) knots 3 3 3 3 4 4 4 4
  line L0 (36.2562, -16.6632) -> (38.4332, -16.6632)
  line L1 (36.2562, -9.0984) -> (36.2562, -16.6632)
  line L2 (38.4332, -16.6632) -> (38.4332, -11.169)
  line L3 (38.4332, -11.169) -> (36.2562, -9.0984)
  spline S2 degree 3 poles (40.7756, -0.0588) (40.7504, -1.4892) (39.5165, -2.6401) (38.093, -2.5986) knots 3 3 3 3 4 4 4 4
  spline S3 degree 3 poles (52.3299, 10.7418) (52.2061, 10.7892) (52.0161, 10.6725) (51.8538, 10.5728) knots 0 0 0 0 1 1 1 1
  ellipse E0 centre (52.1671, 9.9556) end of major axis (53.024, 10.5575) minor radius 0.6882 (51.8538, 10.5728) -> (51.6391, 10.4148) ccw
  line L4 (51.6391, 10.4148) -> (42.645, 3.0208)
  line L5 (42.645, 3.0208) -> (43.5187, 5.4833)
  spline S4 degree 3 poles (43.5187, 5.4833) (43.5384, 5.5707) (43.5881, 5.8447) (43.4359, 6.1071) knots 4 4 4 4 5 5 5 5
  ellipse E1 centre (42.2348, 5.4279) end of major axis (43.445, 6.091) minor radius 1.027 (43.4359, 6.1071) -> (43.2716, 6.3054) ccw
  line L6 (43.2716, 6.3054) -> (37.8047, 12.8944)
  spline S5 degree 3 poles (37.8047, 12.8944) (37.6982, 12.9754) (37.5165, 13.0902) (37.2665, 13.1452) knots 7 7 7 7 8 8 8 8
  ellipse E2 centre (36.8981, 11.5347) end of major axis (36.47, 9.9388) minor radius 1.4889 (37.2665, 13.1452) -> (36.9442, 13.1762) ccw
  line L7 (36.9442, 13.1762) -> (26.9091, 14.0414)
  spline S6 degree 3 poles (26.9091, 14.0414) (26.6003, 14.0294) (26.4058, 13.8151) (26.4226, 13.6428) (26.4379, 13.486) (26.6253, 13.3919) (26.6455, 13.3821) knots 10 10 10 10 11 11 11 12 12 12 12
  line L8 (26.6455, 13.3821) -> (34.9627, 4.0059)
  spline S7 degree 3 poles (34.9627, 4.0059) (33.9839, 4.3564) (33.005, 4.7068) (32.0262, 5.0573) knots 13 13 13 13 14 14 14 14
  spline S8 degree 3 poles (32.0262, 5.0573) (31.987, 5.0654) (31.816, 5.0965) (31.6909, 4.9918) knots 14 14 14 14 15 15 15 15
  ellipse E3 centre (32.6828, 3.8038) end of major axis (33.6744, 2.6156) minor radius 0.6791 (31.6909, 4.9918) -> (31.634, 4.9286) ccw
  line L9 (31.634, 4.9286) -> (26.2858, -1.0117)
  ellipse E4 centre (28.6846, -1.8844) end of major axis (31.2825, -2.3147) minor radius 1.5458 (26.2858, -1.0117) -> (26.0912, -1.4291) ccw
  arc A2 (26.0912, -1.4291) -> (26.0804, -1.4987) centre (26.9815, -1.6026) ccw
  line L10 (26.0804, -1.4987) -> (25.0384, -11.873)
  spline S9 degree 3 poles (25.0384, -11.873) (25.0303, -12.14) (25.1188, -12.3317) (25.2185, -12.3466) knots 20 20 20 20 21 21 21 21
  spline S10 degree 3 poles (25.2185, -12.3466) (25.2902, -12.3573) (25.3947, -12.281) (25.4122, -12.2682) knots 21 21 21 21 22 22 22 22
  ellipse E5 centre (25.1533, -11.8796) end of major axis (25.1612, -12.353) minor radius 0.452 (25.4122, -12.2682) -> (25.5112, -12.1694) ccw
  line L11 (25.5112, -12.1694) -> (33.9632, -3.7207)
  line L12 (33.9632, -3.7207) -> (33.1563, -5.9289)
  spline S11 degree 3 poles (33.1563, -5.9289) (33.1499, -5.9496) (33.1138, -6.0744) (33.186, -6.1783) knots 25 25 25 25 26 26 26 26
  ellipse E6 centre (33.5553, -5.9318) end of major axis (33.93, -5.6937) minor radius 0.3244 (33.186, -6.1783) -> (33.2571, -6.2458) ccw
  line L13 (33.2571, -6.2458) -> (36.2562, -9.0984)
  line L14 (36.2562, -9.0984) -> (38.4332, -11.169)
  line L15 (38.4332, -11.169) -> (39.3848, -12.0741)
  spline S12 degree 3 poles (39.3848, -12.0741) (39.4553, -12.1515) (39.6204, -12.3094) (39.8728, -12.3529) (39.9401, -12.3645) (40.002, -12.366) (40.056, -12.3626) knots 30 30 30 30 31 31 31 32 32 32 32
  line L16 (40.056, -12.3626) -> (47.4062, -12.2645)
  spline S13 degree 3 poles (47.4062, -12.2645) (47.5967, -12.2807) (47.7724, -12.2098) (47.8393, -12.0798) knots 33 33 33 33 34 34 34 34
  spline S14 degree 3 poles (47.8393, -12.0798) (47.9186, -11.9256) (47.8231, -11.7307) (47.7691, -11.6206) knots 34 34 34 34 35 35 35 35
  ellipse E7 centre (47.217, -11.8532) end of major axis (47.6137, -12.4472) minor radius 0.5959 (47.7691, -11.6206) -> (47.6862, -11.4851) ccw
  line L17 (47.6862, -11.4851) -> (41.6732, -4.6814)
  line L18 (41.6732, -4.6814) -> (43.0967, -5.1971)
  spline S15 degree 3 poles (43.0967, -5.1971) (43.1354, -5.2175) (43.3177, -5.3084) (43.5239, -5.2382) knots 38 38 38 38 39 39 39 39
  spline S16 degree 3 poles (43.5239, -5.2382) (43.6184, -5.206) (43.6833, -5.1518) (43.7205, -5.1144) knots 39 39 39 39 40 40 40 40
  spline S17 degree 3 poles (43.7205, -5.1144) (43.6772, -5.1417) (49.8217, -1.28) (49.8217, -1.28) knots 40 40 40 40 41 41 41 41
  spline S18 degree 3 poles (49.8217, -1.28) (49.956, -1.2027) (50.3034, -0.9774) (50.4312, -0.5559) knots 41 41 41 41 42 42 42 42
  ellipse E8 centre (47.3975, 0.3569) end of major axis (50.4322, -0.5527) minor radius 1.8585 (50.4312, -0.5559) -> (50.4774, -0.2866) ccw
  line L19 (50.4774, -0.2866) -> (52.4779, 10.0091)
  spline S19 degree 3 poles (52.4779, 10.0091) (52.5499, 10.3808) (52.4796, 10.6846) (52.3299, 10.7418) knots 44 44 44 44 45 45 45 45
  circle A3 centre (38.1897, -0.0141) radius 2.5863
  circle A4 centre (38.2989, -0.3433) radius 5.4959 construction
  dimension "d163" = 18
  dimension "d164" = 1.5
  constraint coincident A0.centre A1.centre
  constraint concentric A0 A1
  constraint coincident S1.end A3
  constraint coincident S0.end A3
  constraint coincident S0.start A3
  constraint coincident L11.end A4
  constraint coincident L17.end A4
  constraint coincident L4.end A4
  measures "d163" diameter of A0
  measures "d164" distance of A0 A1
extrude "Extrusão1''''''" add sketch "Esboço1 (8)" along normal blind 13.5 separate body contours A0 makes body 8 in component "Peça_Disco"
extrude "Extrusão2''''''" add sketch "Esboço1 (8)" along normal blind 12 contours A1 bodies 8 in component "Peça_Disco"
move_body "Mover1" bodies 8 to x (1, 0, 0) y (0, 1, 0) z (0, 0, 1) at (0, 0, 100) in component "Peça_Disco"
other "Organizar1"
other "Organizar2"
component "Camada_2" placed x (1, 0, 0) y (0, 1, 0) z (0, 0, 1) at (0, 0, 0)
component "Camada_3" placed x (1, 0, 0) y (0, 1, 0) z (0, 0, 1) at (0, 0, 0)
component "Camada_4" placed x (1, 0, 0) y (0, 1, 0) z (0, 0, 1) at (0, 0, 0)
component "Base" placed x (1, 0, 0) y (0, 1, 0) z (0, 0, 1) at (0, 0, 0)
component "Tampa_cam1" placed x (1, 0, 0) y (0, 1, 0) z (0, 0, 1) at (0, 0, 0)
component "Eixo_1" placed x (1, 0, 0) y (0, 1, 0) z (0, 0, 1) at (0, 0, 0)
component "Eixo_2" placed x (1, 0, 0) y (0, 1, 0) z (0, 0, 1) at (0, 0, 0)
component "Peça_Disco" placed x (1, 0, 0) y (0, 1, 0) z (0, 0, 1) at (0, 0, 0)
component "Organizar1" placed x (1, 0, 0) y (0, 1, 0) z (0, 0, 1) at (0, 0, 0)
component "Organizar2" placed x (1, 0, 0) y (0, 1, 0) z (0, 0, 1) at (0, 0, 0)
component "Invólucro1(Qtd: 1)" placed x (0, 0, 1) y (1, 0, 0) z (0, 1, 0) at (100, 0, 0) in component "Organizar1"
component "Camada_2" placed x (0, 1, 0) y (0, 0, -1) z (-1, 0, 0) at (183.7, 86.6339, 70) in component "Invólucro1(Qtd: 1)"
component "Camada_3" placed x (0, -1, 0) y (0, 0, -1) z (1, 0, 0) at (295.3723, 131.5228, 50) in component "Invólucro1(Qtd: 1)"
component "Camada_4" placed x (0, -1, 0) y (0, 0, -1) z (1, 0, 0) at (63.35, 110.573, 30) in component "Invólucro1(Qtd: 1)"
component "Base" placed x (0, 1, 0) y (0, 0, 1) z (1, 0, 0) at (397.4, 63.35, 0) in component "Invólucro1(Qtd: 1)"
component "Eixo_1" placed x (0, 1, 0) y (-1, 0, 0) z (0, 0, 1) at (334.05, 35.662, 5) in component "Invólucro1(Qtd: 1)"
component "Eixo_2" placed x (0, 0, 1) y (1, 0, 0) z (0, 1, 0) at (358.7223, 136.7, 5) in component "Invólucro1(Qtd: 1)"
component "Peça_Disco" placed x (1, 0, 0) y (0, 0, 1) z (0, -1, 0) at (255.9296, 168.6471, 0) in component "Invólucro1(Qtd: 1)"
component "Invólucro1(Qtd: 1) (1)" placed x (0, 0, 1) y (1, 0, 0) z (0, 1, 0) at (360, 0, 0) in component "Organizar2"
component "Tampa_cam1" placed x (0, 1, 0) y (0, 0, -1) z (-1, 0, 0) at (63.35, 63.35, 90) in component "Invólucro1(Qtd: 1) (1)"
equation "Exp_fina = 10 mm" comment "Para o eixo"
equation "Exp_grossa = 20 mm" comment "Peça giratória e base (camadas?)"
equation "Eixo_larg = 20 mm"
equation "Eixo_comp = 90 mm" comment "Altura do objeto"
equation "Gira_diam = Eixo_larg + 0.5 mm" comment "Expessura fina mais folga, para a peça poder girar"
equation "Gira_grossura = 7 mm" comment "Grossura da peça giratória"
equation "Gira_comp = Gira_diam + Gira_grossura + 4 mm"
equation "Peça_diam = Eixo_larg + Gira_grossura + Gira_grossura + 80 mm" comment "Tem q dar 12."
equation "Borda = 5 mm" comment "Para o berlinde não cair"
equation "Disco_comp = 18 mm" comment "Comprimento da peça disco"
equation "Aperto = 0.2 mm"
equation "Disco_buraco = 20 mm" comment "Buraco para o disco"
equation "Exp_minima = 5 mm"
equation "Disco_alt = 13.5 mm" comment "Altura da peça disco"
equation "Exp_fan = 3 mm" comment "expessura das pás da ventoinha"
equation "d39 = Exp_fina"
equation "d40 = Exp_fina"
equation "d41 = Eixo_larg"
equation "d42 = Eixo_larg"
equation "d43 = Aperto"
equation "d45 = Peça_diam"
equation "d46 = Borda"
equation "d47 = Exp_fan"
equation "d48 = Disco_buraco"
equation "d49 = Disco_buraco"
equation "d50 = Disco_buraco"
equation "d51 = Peça_diam / 4 + Exp_minima / 2"
equation "d52 = Disco_buraco"
equation "d53 = Disco_buraco"
equation "d54 = Disco_buraco"
equation "d55 = Peça_diam / 4 + Borda / 2"
equation "d56 = Exp_minima * 2"
equation "d58 = Exp_minima"
equation "d61 = Exp_grossa"
equation "d64 = -Exp_minima"
equation "d67 = -Exp_minima - Borda"
equation "d70 = -Exp_minima - Exp_fan"
equation "d73 = Exp_grossa"
equation "d76 = -Exp_minima"
equation "d79 = -Exp_minima - Borda"
equation "d82 = -Exp_fan"
equation "d85 = Exp_grossa"
equation "d88 = -Exp_minima"
equation "d91 = -Borda"
equation "d94 = -Exp_fan"
equation "d97 = Exp_grossa"
equation "d100 = -Exp_minima"
equation "d103 = -Borda"
equation "d106 = -Exp_fan"
equation "d112 = Exp_fina"
equation "d113 = Eixo_comp / 2"
equation "Fresa_bones = 3 mm" comment "tamanho da fresampara cortar"
equation "d117 = Fresa_bones"
equation "d118 = Fresa_bones"
equation "d119 = Exp_fina"
equation "d120 = Eixo_comp / 2"
equation "d121 = Fresa_bones"
equation "d122 = Fresa_bones"
equation "d163 = Disco_comp"
equation "d164 = Exp_fan / 2"
equation "d166 = Disco_alt"
equation "d168 = Disco_alt - Exp_fan / 2"
